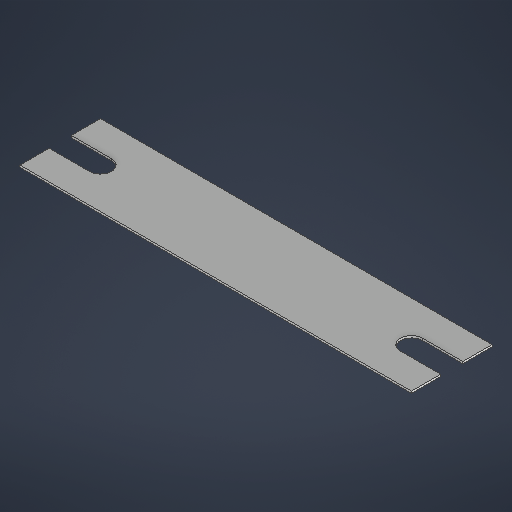
# Autodesk Inventor part: Galvo Spacer Y
Saved by Autodesk Inventor 2025 (Build 290162000, 162)
## iProperties
Created: 2024-07-08
Part Number: Galvo Spacer Y
Material: Generic
Document SubType Name: Modeling
Designer: mayhe
Density: 1 g/cm^3
Appearance: Default
Author: mayhe
Autodesk Inventor part; units mm, degrees
ref_plane "YZ Plane" through (0, 0, 0) normal (1, 0, 0) x (0, 1, 0)
ref_plane "XZ Plane" through (0, 0, 0) normal (0, 1, 0) x (-1, 0, 0)
ref_plane "XY Plane" through (0, 0, 0) normal (0, 0, 1) x (1, 0, 0)
sketch "Sketch5" plane through (0, 0, 0) normal (0, 0, 1) x (1, 0, 0)
  line L0 (68.6, -0.25) -> (-28.6, -0.25)
  line L1 (-28.6, -0.25) -> (-28.6, 0.25)
  line L2 (-28.6, 0.25) -> (68.6, 0.25)
  line L3 (68.6, 0.25) -> (68.6, -0.25)
  line L4 (68.6, -0.25) -> (-28.6, 0.25) construction
  line L5 (-28.6, -0.25) -> (68.6, 0.25) construction
  point P0 (20, 0)
  dimension "d83" = 97.2
  dimension "d84" = 0.5
  constraints: 12 end point, 2 midpoint, 2 parallel, 1 horizontal, 1 perpendicular
  measures "d83" distance of L1.end L2.end
  measures "d84" distance of L0.end L1.end
extrude "Extrusion5" add sketch "Sketch5" along normal mid plane 20
sketch "Sketch7" plane through (-28.6, -0.25, 10) normal (0, -1, 0) x (1, 0, 0)
  circle A0 centre (87.2, -10) radius 2.75
  circle A1 centre (10, -10) radius 2.75
  line L0 (0, 0) -> (97.2, 0) projected
  line L1 (97.2, -20) -> (97.2, 0) projected
  line L2 (0, -20) -> (0, 0) projected
  line L3 (87.2, -12.75) -> (97.2, -12.75)
  line L4 (97.2, -12.75) -> (97.2, -7.25)
  line L5 (97.2, -7.25) -> (87.2, -7.25)
  line L6 (87.2, -7.25) -> (87.2, -12.75)
  line L7 (10, -12.75) -> (0, -12.75)
  line L8 (0, -12.75) -> (0, -7.25)
  line L9 (0, -7.25) -> (10, -7.25)
  line L10 (10, -7.25) -> (10, -12.75)
  point P0 (28.6, -10)
  point P1 (0, -10)
  dimension "d85" = 5.5
  dimension "d86" = 5.5
  dimension "d87" = 10
  dimension "d88" = 10
  dimension "d89" = 10
  dimension "d90" = 10
  constraints: 16 end point, 4 parallel, 4 point on line, 2 horizontal, 2 perpendicular, 1 midpoint, 6 other
  measures "d87" distance from line of L0 point (87.2, -10)
  measures "d88" distance from line of L1 point (87.2, -10)
  measures "d89" distance of point (0, -10) point (10, -10)
  measures "d90" distance from line of L0 point (10, -10)
extrude "Extrusion7" cut sketch "Sketch7" against normal blind 20
body "Solid3"
